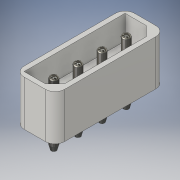
# Autodesk Inventor part: Molex_4x508_Conn
Saved by Autodesk Inventor 2016 (Build 200138000, 138)
## iProperties
Created: 2016-09-02
Part Number: Molex_4x508_Conn
Material: Generic
Document SubType Name: Modeling
Designer: jfixelle
Density: 1 g/cm^3
Appearance: White
Author: jfixelle
Autodesk Inventor part; units mm, degrees
ref_plane "YZ Plane" through (0, 0, 0) normal (1, 0, 0) x (0, 1, 0)
ref_plane "XZ Plane" through (0, 0, 0) normal (0, 1, 0) x (-1, 0, 0)
ref_plane "XY Plane" through (0, 0, 0) normal (0, 0, 1) x (1, 0, 0)
sketch "Sketch1" plane through (0, 0, 0) normal (0, 1, 0) x (-1, 0, 0)
  line L0 (4.25, 11.62) -> (-4.25, 11.62)
  line L1 (-4.25, 11.62) -> (-4.25, -11.62)
  line L2 (-4.25, -11.62) -> (4.25, -11.62)
  line L3 (4.25, -11.62) -> (4.25, 11.62)
  point P0 (0, 0)
  dimension "d0" = 23.24
  dimension "d1" = 11.62
  dimension "d2" = 8.5
  dimension "d3" = 4.25
  constraints: 8 end point, 2 parallel, 1 horizontal, 1 perpendicular
  measures "d0" distance of L2.end L0.start
  measures "d1" distance from line of L2 point (0, 0)
  measures "d2" distance of L1.end L2.end
  measures "d3" distance from line of point (0, 0) L3
extrude "Extrusion1" add sketch "Sketch1" along normal blind 9.53
fillet "Fillet1" radius 2 4 edges at (4.25, 4.765, 11.62) (-4.25, 4.765, 11.62) (-4.25, 4.765, -11.62) (4.25, 4.765, -11.62)
sketch "Sketch2" plane through (0, 9.53, 0) normal (0, 1, 0) x (1, 0, 0)
  line L0 (-3.25, -10.62) -> (3.25, -10.62)
  line L1 (3.25, -10.62) -> (3.25, 10.62)
  line L2 (3.25, 10.62) -> (-3.25, 10.62)
  line L3 (-3.25, 10.62) -> (-3.25, -10.62)
  line L4 (4.25, 11.62) -> (-4.25, 11.62) projected
  line L5 (-4.25, 11.62) -> (-4.25, -11.62) projected
  line L6 (-4.25, -11.62) -> (4.25, -11.62) projected
  line L7 (4.25, -11.62) -> (4.25, 11.62) projected
  line L8 (1.25, 10.62) -> (3.25, 8.62)
  line L9 (3.25, -8.62) -> (1.25, -10.62)
  point P0 (0, 0)
  dimension "d6" = 1
  dimension "d7" = 1
  dimension "d8" = 1
  dimension "d9" = 1
  dimension "d11" = 45
  dimension "d12" = 45
  dimension "d13" = 2
  dimension "d14" = 2
  constraints: 12 end point, 4 point on line, 2 parallel, 1 horizontal, 1 perpendicular
  measures "d6" distance between parallel lines of L4 L2
  measures "d7" distance between parallel lines of L3 L5
  measures "d8" distance between parallel lines of L6 L0
  measures "d9" distance between parallel lines of L7 L1
  measures "d11" angle of L1 L8
  measures "d12" angle of L1 L9
  measures "d13" distance from line of L1 L9.end
  measures "d14" distance from line of L1 L8.start
extrude "Extrusion2" cut sketch "Sketch2" against normal blind 5.08 contours L3 L2 L8 L1 L9 L0
sketch "Sketch3" plane through (0, 0, 0) normal (0, -1, 0) x (1, 0, 0)
  circle A0 centre (0, 7.62) radius 0.8
  point P0 (0, 0)
  dimension "d17" = 1.6
  dimension "d18" = 7.62
  constraints: 1 centre point
  measures "d17" diameter of A0
  measures "d18" distance of point (0, 0) A0.centre
extrude "Extrusion3" add sketch "Sketch3" along normal blind 4.57 and the other way blind 8.89
fillet "Fillet2" radius 0.508 1 edges at (-0.8, 8.89, 7.62)
chamfer "Chamfer1" distance 1 angle 15 1 edges at (-0.8, -4.57, 7.62) measured on face at (0.7974, -3.0467, 7.5556)
pattern_linear "Rectangular Pattern1" count 4 spacing 5.08 along (0, 0, -1) of "Extrusion3", "Fillet2", "Chamfer1"
body "Solid1"
